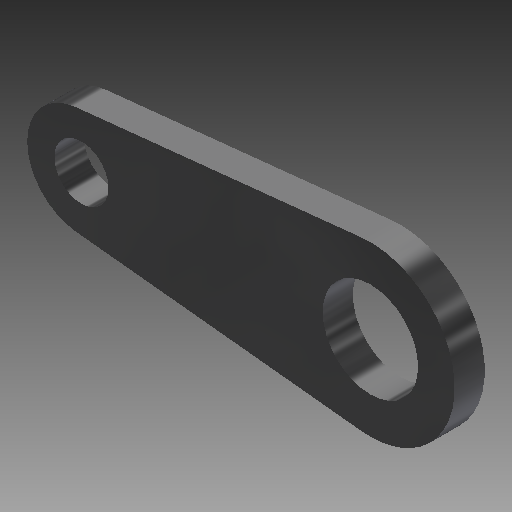
# Autodesk Inventor part: 313-01-03
Saved by Autodesk Inventor 2019 (Build 230136000, 136)
## iProperties
Company: Autodesk Inc.
Created: 2007-10-25
Part Number: 313-01-03
Document SubType Name: Modeling
Designer: Autodesk Inc.
Density: 7.85 g/cm^3
Mass: 50.4138 g
Surface Area: 38.0293 cm^2
Volume: 6.42214 cm^3
Material: Steel
Description: PIVOT PLATE - REAR
Appearance: Rubber - Black - Version 1.1
Component Category: Lower Component
Author: Inventor
Autodesk Inventor part; units mm, degrees
ref_plane "YZ Plane" through (0, 0, 0) normal (1, 0, 0) x (0, 1, 0)
ref_plane "XZ Plane" through (0, 0, 0) normal (0, 1, 0) x (-1, 0, 0)
sketch "Sketch1" plane through (0, 0, 0) normal (0, 0, 1) x (1, 0, 0)
  circle A0 centre (0, 0) radius 14
  line L0 (0, 0) -> (-48, 0) construction
  circle A1 centre (-48, 0) radius 9
  line L1 (-48.9375, 8.951) -> (-1.4583, 13.9238)
  line L2 (-48.9375, -8.951) -> (-1.4583, -13.9238)
  dimension "d0" = 18
  dimension "d1" = 28
  dimension "d2" = 48
  constraints: 6 end point, 4 point on circle, 4 tangent, 2 centre point, 2 coincident, 1 horizontal
  measures "d0" diameter of A1
  measures "d1" diameter of A0
  measures "d2" distance of point (0, 0) L0.end
extrude "Extrusion1" add sketch "Sketch1" along normal mid plane 5
sketch "Sketch2" plane through (0, 0, 2.5) normal (0, 0, 1) x (1, 0, 0)
  arc A0 (-1.4583, -13.9238) -> (-1.4583, 13.9238) centre (0, 0) ccw projected
hole "Hole1" at (0, 0, 2.5) direction (0, 0, -1) diameter 15.84 end through all
sketch "Sketch3" plane through (0, 0, 2.5) normal (0, 0, 1) x (1, 0, 0)
  arc A0 (-48.9375, 8.951) -> (-48.9375, -8.951) centre (-48, 0) ccw projected
hole "Hole2" at (-48, 0, 2.5) direction (0, 0, -1) diameter 9 end through all
body "Solid1"
